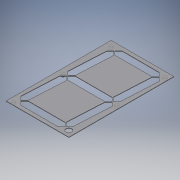
# Autodesk Inventor part: Cover-7-Segment
Saved by Autodesk Inventor 2016 SP2 (Build 200236200, 236)
## iProperties
Created: 2018-06-10
Part Number: Cover-7-Segment
Material: Generisch
Document SubType Name: Modeling
Designer: Nils
Density: 1 g/cm^3
Appearance: Vorgabe
Author: Nils
Autodesk Inventor part; units mm, degrees
ref_plane "YZ Plane" through (0, 0, 0) normal (1, 0, 0) x (0, 1, 0)
ref_plane "XZ Plane" through (0, 0, 0) normal (0, 1, 0) x (-1, 0, 0)
ref_plane "XY Plane" through (0, 0, 0) normal (0, 0, 1) x (1, 0, 0)
sketch "Skizze1" plane through (0, 0, 0) normal (0, 0, 1) x (1, 0, 0)
  line L0 (0, 0) -> (85.2336, 0)
  line L1 (85.2336, 0) -> (85.2336, 142.6914)
  line L2 (85.2336, 142.6914) -> (0, 142.6914)
  line L3 (0, 142.6914) -> (0, 0)
  circle A0 centre (77.2336, 8) radius 4
  line L4 (20.2336, 137.6914) -> (15.2336, 132.6914)
  line L5 (15.2336, 132.6914) -> (20.2336, 127.6914)
  line L6 (20.2336, 127.6914) -> (70.2336, 127.6914)
  line L7 (70.2336, 127.6914) -> (75.2336, 132.6914)
  line L8 (75.2336, 132.6914) -> (70.2336, 137.6914)
  line L9 (70.2336, 137.6914) -> (20.2336, 137.6914)
  line L10 (14.5265, 131.9843) -> (19.5265, 126.9843)
  line L11 (19.5265, 126.9843) -> (16.9097, 77.0528)
  line L12 (16.9097, 77.0528) -> (11.9097, 72.0528)
  line L13 (11.9097, 72.0528) -> (6.9097, 77.0528)
  line L14 (6.9097, 77.0528) -> (9.5265, 126.9843)
  line L15 (9.5265, 126.9843) -> (14.5265, 131.9843)
  line L16 (75.9407, 131.9843) -> (80.9407, 126.9843)
  line L17 (80.9407, 126.9843) -> (78.3239, 77.0528)
  line L18 (78.3239, 77.0528) -> (73.3239, 72.0528)
  line L19 (73.3239, 72.0528) -> (68.3239, 77.0528)
  line L20 (68.3239, 77.0528) -> (70.9407, 126.9843)
  line L21 (70.9407, 126.9843) -> (75.9407, 131.9843)
  line L22 (11.9097, 70.6386) -> (6.9097, 65.6386)
  line L23 (6.9097, 65.6386) -> (4.2929, 15.7071)
  line L24 (4.2929, 15.7071) -> (9.2929, 10.7071)
  line L25 (9.2929, 10.7071) -> (14.2929, 15.7071)
  line L26 (14.2929, 15.7071) -> (16.9097, 65.6386)
  line L27 (16.9097, 65.6386) -> (11.9097, 70.6386)
  line L28 (12.6168, 71.3457) -> (17.6168, 76.3457)
  line L29 (17.6168, 76.3457) -> (67.6168, 76.3457)
  line L30 (67.6168, 76.3457) -> (72.6168, 71.3457)
  line L31 (72.6168, 71.3457) -> (67.6168, 66.3457)
  line L32 (67.6168, 66.3457) -> (17.6168, 66.3457)
  line L33 (17.6168, 66.3457) -> (12.6168, 71.3457)
  line L34 (15, 15) -> (65, 15)
  line L35 (65, 15) -> (70, 10)
  line L36 (70, 10) -> (65, 5)
  line L37 (65, 5) -> (15, 5)
  line L38 (15, 15) -> (10, 10)
  line L39 (10, 10) -> (15, 5)
  line L40 (70.7071, 10.7071) -> (65.7071, 15.7071)
  line L41 (65.7071, 15.7071) -> (68.3239, 65.6386)
  line L42 (68.3239, 65.6386) -> (73.3239, 70.6386)
  line L43 (73.3239, 70.6386) -> (78.3239, 65.6386)
  line L44 (78.3239, 65.6386) -> (75.7071, 15.7071)
  line L45 (75.7071, 15.7071) -> (70.7071, 10.7071)
  dimension "d24" = 8
  dimension "d25" = 8
  dimension "d26" = 8
  dimension "d27" = 5
  dimension "d28" = 10
  dimension "d30" = 1
  dimension "d31" = 3
  dimension "d32" = 0
  dimension "d33" = 10
  dimension "d34" = 135
  dimension "d35" = 1
  dimension "d36" = 0
  dimension "d37" = 1
  dimension "d38" = 0
  dimension "d39" = 1
  dimension "d40" = 0
  dimension "d41" = 1
  dimension "d42" = 5
  dimension "d43" = 10
  dimension "d44" = 1
  dimension "d45" = 1
  dimension "d48" = 50
  dimension "d49" = 85.2336
  dimension "d50" = 142.6914
  constraints: 92 end point, 58 equal length, 9 perpendicular, 4 horizontal, 1 centre point, 1 point on line
  measures "d24" diameter of A0
  measures "d25" distance from line of L1 A0.centre
  measures "d26" distance from line of L0 A0.centre
  measures "d27" distance between parallel lines of L0 L37
  measures "d28" distance from line of L3 L38.end
  measures "d30" distance between parallel lines of L38 L25
  measures "d31" angle of L3 L23
  measures "d32" distance between parallel lines of L24 L39
  measures "d33" distance between parallel lines of L34 L37
  measures "d34" angle of L37 L39
  measures "d35" distance between parallel lines of L33 L27
  measures "d36" distance between parallel lines of L22 L28
  measures "d37" distance between parallel lines of L19 L30
  measures "d38" distance between parallel lines of L18 L31
  measures "d39" distance between parallel lines of L28 L12
  measures "d40" distance between parallel lines of L33 L13
  measures "d41" distance between parallel lines of L10 L5
  measures "d42" distance between parallel lines of L2 L9
  measures "d43" distance from line of L1 L7.end
  measures "d44" distance between parallel lines of L42 L31
  measures "d45" distance between parallel lines of L43 L19
  measures "d48" distance of L36.end L37.end
  measures "d49" distance of L1.end L2.end
  measures "d50" distance of L0.end L1.end
extrude "Extrusion1" add sketch "Skizze1" along normal blind 0.6
sketch "Skizze3" plane through (0, 0, 0) normal (0, 0, -1) x (-1, 0, 0)
  circle A0 centre (-79.2336, 71.3457) radius 2.5 construction
  circle A1 centre (-5, 5) radius 2.5 construction
  circle A2 centre (-6, 71.3457) radius 2.5 construction
  circle A3 centre (-6, 136.6914) radius 2.5 construction
  circle A4 centre (-79.2336, 136.6914) radius 2.5 construction
  circle A5 centre (-79.2336, 136.6914) radius 2.4
  circle A6 centre (-6, 136.6914) radius 2.4
  circle A7 centre (-79.2336, 71.3457) radius 2.4
  circle A8 centre (-6, 71.3457) radius 2.4
  circle A9 centre (-5, 5) radius 2.4
  point P0 (0, 0)
  dimension "d51" = 4.8
  dimension "d52" = 4.8
  dimension "d53" = 4.8
  dimension "d54" = 4.8
  dimension "d55" = 4.8
  constraints: 5 centre point, 5 coincident
  measures "d51" diameter of A5
  measures "d52" diameter of A6
  measures "d53" diameter of A7
  measures "d54" diameter of A8
  measures "d55" diameter of A9
extrude "Extrusion2" add sketch "Skizze3" along normal blind 2.5
